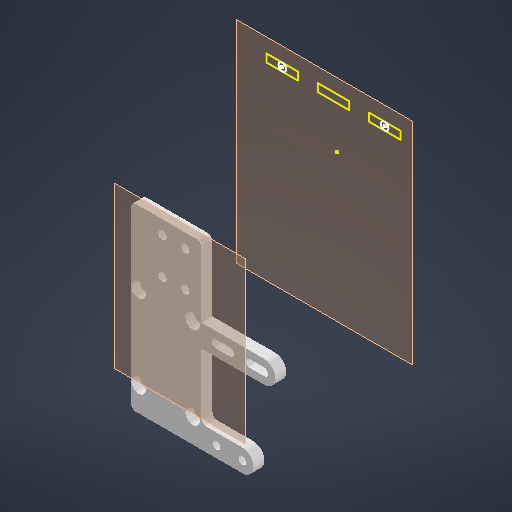
# Autodesk Inventor part: rails-bolts
Saved by Autodesk Inventor 2025 (Build 290162000, 162)
## iProperties
Created: 2024-07-18
Part Number: rails-bolts
Material: Generic
Document SubType Name: Modeling
Designer: Windows 7 was better
Density: 1 g/cm^3
Appearance: Default
Author: Windows 7 was better
Autodesk Inventor part; units mm, degrees
ref_plane "YZ Plane" through (0, 0, 0) normal (1, 0, 0) x (0, 1, 0)
ref_plane "XZ Plane" through (0, 0, 0) normal (0, 1, 0) x (-1, 0, 0)
ref_plane "XY Plane" through (0, 0, 0) normal (0, 0, 1) x (1, 0, 0)
ref_plane "Work Plane1" through (-1.6596, -28.9901, 28.1919) normal (0, 0, 1) x (1, 0, 0)
sketch "Sketch1" plane through (-1.6596, -28.9901, 28.1919) normal (0, 0, 1) x (1, 0, 0)
  circle A0 centre (-7.0449, 11.8967) radius 1.75 projected
  circle A1 centre (2.3051, 12.2717) radius 1.75 projected
  circle A2 centre (2.3051, 26.8467) radius 1.75 projected
  circle A3 centre (-7.0449, 26.8467) radius 1.75 projected
  line L0 (2.3051, 26.8467) -> (2.3051, 32.4467) construction
  line L1 (2.3051, 32.4467) -> (-7.0449, 32.4467) construction
  line L2 (-7.0449, 32.4467) -> (-7.0449, 26.8467) construction
  spline S0 degree 3 poles (-18.1261, -96.0287) (-18.1261, -96.0287) (-18.0932, -96.0287) (-18.0298, -96.0287) (-17.8251, -96.0287) (-17.2794, -96.0287) (-16.7467, -96.0287) (-16.213, -96.0287) (-15.7353, -96.0287) (-15.6244, -96.0287) (-15.6063, -96.0287) (-15.5971, -96.0287) (-15.5971, -96.0287) knots 0.499993 0.499993 0.499993 0.499993 0.562494 0.562494 0.562494 0.764477 0.764477 0.764477 0.966846 0.966846 0.966846 1 1 1 1 construction
  line L3 (-18.3185, -96.0287) -> (-15.9665, -96.0287) construction
  arc A4 (-13.8616, 2.5089) -> (-19.8616, 2.5089) centre (-16.8616, 2.5089) ccw construction
  arc A5 (-13.9993, -31.5037) -> (-19.9993, -31.5037) centre (-16.9993, -31.5037) ccw construction
  arc A6 (3.0015, -1.5044) -> (9.0015, -1.5044) centre (6.0015, -1.5044) ccw
  line L4 (-19.9993, 32.4467) -> (9.0007, 32.4467)
  line L5 (9.0007, 32.4467) -> (9.0007, -34.5533)
  line L6 (9.0007, -34.5533) -> (-19.9993, -34.5533)
  line L7 (-19.9993, -34.5533) -> (-19.9993, 32.4467)
  circle A7 centre (-16.8616, -31.5037) radius 1.6
  circle A8 centre (5.3371, -31.5037) radius 1.6
  circle A9 centre (-16.8616, 2.5089) radius 1.6
  circle A10 centre (5.3371, 2.5089) radius 1.6
  point P0 (1.6596, 28.9901)
  point P1 (-18.3185, 3.0171)
  point P2 (-15.9662, 3.4042)
  dimension "d0" = 5.6
  dimension "d1" = 29
  dimension "d2" = 67
  dimension "d5" = 3.2
  dimension "d6" = 3.2
  dimension "d7" = 3.2
  dimension "d8" = 3.2
  constraints: 16 end point, 7 centre point, 6 point on circle, 3 perpendicular, 2 horizontal, 2 parallel, 1 coincident, 1 vertical, 20 other
  measures "d0" distance of L0.start L0.end
  measures "d1" distance of L5.end L6.end
  measures "d2" distance of L4.end L5.end
  measures "d5" diameter of A7
  measures "d6" diameter of A8
  measures "d7" diameter of A9
  measures "d8" diameter of A10
ref_plane "Work Plane2" through (-8.6352, -23.8919, -35.0523) normal (0, 0, 1) x (1, 0, 0)
sketch "Sketch2" plane through (-8.6352, -23.8919, -35.0523) normal (0, 0, 1) x (1, 0, 0)
  line L0 (-7.5414, 41.3535) -> (-20.5414, 41.3535) projected
  line L1 (-20.5414, 44.5535) -> (-7.5414, 44.5535) projected
  line L2 (-7.5414, 44.5535) -> (-7.5414, 41.3535) projected
  line L3 (-20.5414, 41.3535) -> (-20.5414, 44.5535) projected
  line L4 (13.5, 41.3535) -> (0.5, 41.3535) projected
  line L5 (0.5, 44.5535) -> (13.5, 44.5535) projected
  line L6 (13.5, 44.5535) -> (13.5, 41.3535) projected
  line L7 (0.5, 41.3535) -> (0.5, 44.5535) projected
  line L8 (34.55, 41.3535) -> (21.55, 41.3535) projected
  line L9 (21.55, 44.5535) -> (34.55, 44.5535) projected
  line L10 (21.55, 41.3535) -> (21.55, 44.5535) projected
  line L11 (34.55, 44.5535) -> (34.55, 41.3535) projected
  line L12 (-14.0414, 44.5535) -> (-14.0414, 41.3535) construction
  line L13 (28.05, 44.5535) -> (28.05, 41.3535) construction
  circle A0 centre (-14.0414, 42.9535) radius 1.6
  circle A1 centre (28.05, 42.9535) radius 1.6
  point P0 (8.6352, 23.8919)
  constraints: 6 midpoint, 4 end point, 2 vertical alignment, 4 other
extrude "Extrusion1" add sketch "Sketch1" against normal blind 4.5
sketch "Sketch3" plane through (-1.6596, -28.9901, 28.1919) normal (0, 0, 1) x (1, 0, 0)
  line L0 (19.4071, -58.7998) -> (21.4071, -58.7998) construction
  line L1 (20.4071, -58.7998) -> (20.4979, -36.9098) construction
  line L2 (20.4979, -36.9098) -> (25.7879, -36.9098) construction
  line L3 (25.7879, -36.9098) -> (15.2079, -36.9098) construction
  circle A0 centre (15.2079, -36.9098) radius 1.6
  circle A1 centre (25.7879, -36.9098) radius 1.6
  circle A2 centre (15.2079, -36.9098) radius 4.6
  circle A3 centre (25.7879, -36.9098) radius 4.6
  line L4 (25.7879, -32.3098) -> (9.0007, -32.3098)
  line L5 (9.0007, -34.5533) -> (9.0007, 32.4467) projected
  line L6 (25.7879, -41.5098) -> (15.2079, -41.5098)
  line L7 (15.2079, -41.5098) -> (-19.9993, -41.5098)
  line L8 (-19.9993, -34.5533) -> (-19.9993, 32.4467) projected
  line L9 (-19.9993, -41.5098) -> (-19.9993, -34.5533)
  line L10 (-19.9993, -34.5533) -> (9.0007, -34.5533)
  line L11 (9.0007, -34.5533) -> (9.0007, -32.3098)
  line L12 (25.7879, -36.9098) -> (30.1497, -38.3706)
  line L13 (45.9071, 7.0963) -> (8.7371, 7.0963) construction
  line L14 (8.7371, 7.0963) -> (14.7371, 7.0963) construction
  line L15 (14.7371, 7.0963) -> (14.7371, -0.9037) construction
  line L16 (14.7371, -0.9037) -> (34.7371, -0.9037) construction
  line L17 (14.7371, -0.9037) -> (20.7371, -0.9037) construction
  line L18 (14.7371, -2.5037) -> (20.7371, -2.5037)
  line L19 (20.7371, 0.6963) -> (14.7371, 0.6963)
  arc A4 (14.7371, 0.6963) -> (14.7371, -2.5037) centre (14.7371, -0.9037) ccw
  arc A5 (20.7371, -2.5037) -> (20.7371, 0.6963) centre (20.7371, -0.9037) ccw
  line L20 (34.7371, -0.9037) -> (28.7371, -0.9037) construction
  line L21 (34.7371, 0.6963) -> (28.7371, 0.6963)
  line L22 (28.7371, -2.5037) -> (34.7371, -2.5037)
  arc A6 (34.7371, -2.5037) -> (34.7371, 0.6963) centre (34.7371, -0.9037) ccw
  arc A7 (28.7371, 0.6963) -> (28.7371, -2.5037) centre (28.7371, -0.9037) ccw
  line L23 (34.7371, 3.6963) -> (28.7371, 3.6963)
  arc A8 (28.7371, 3.6963) -> (28.7371, -5.5037) centre (28.7371, -0.9037) ccw
  line L24 (28.7371, -5.5037) -> (34.7371, -5.5037)
  arc A9 (34.7371, -5.5037) -> (34.7371, 3.6963) centre (34.7371, -0.9037) ccw
  line L25 (28.7371, 3.6963) -> (9.0007, 3.6963)
  line L26 (28.7371, -5.5037) -> (9.0007, -5.5037)
  point P0 (1.6596, 28.9901)
  point P1 (11.4479, -23.0098)
  point P2 (9.0007, -15.5098)
  point P3 (17.7371, -0.9037)
  point P4 (31.7371, -0.9037)
  dimension "d9" = 10.58
  dimension "d10" = 5.29
  dimension "d11" = 10.58
  dimension "d12" = 3.2
  dimension "d13" = 3.2
  dimension "d14" = 3
  dimension "d15" = 3
  dimension "d43" = 6
  dimension "d44" = 8
  dimension "d45" = 20
  dimension "d46" = 6
  dimension "d47" = 3.2
  dimension "d48" = 6
  dimension "d49" = 3.2
  dimension "d50" = 3
  constraints: 54 end point, 15 point on circle, 9 centre point, 9 tangent, 8 point on line, 7 perpendicular, 5 horizontal, 4 parallel, 3 midpoint, 2 coincident, 1 collinear, 1 vertical alignment, 12 other
  measures "d9" distance of L3.end L2.end
  measures "d10" distance of L1.end L2.end
  measures "d11" distance of L2.end L3.end
  measures "d12" diameter of A0
  measures "d13" diameter of A1
  measures "d15" radial gap between concentric circles of A1 A3
  measures "d43" distance of L13.end L14.end
  measures "d44" distance of L14.end L15.end
  measures "d45" distance of L15.end L16.end
  measures "d46" distance of L15.end L17.end
  measures "d47" diameter of A5
  measures "d48" distance of L16.end L20.end
  measures "d49" diameter of A7
  measures "d50" radial gap between concentric circles of A6 A9
extrude "Extrusion2" add sketch "Sketch3" against normal blind 4.5
sketch "Sketch4" plane through (-1.6596, -28.9901, 23.6919) normal (0, 0, -1) x (-1, 0, 0)
  circle A0 centre (-2.3051, 26.8467) radius 1.75 projected
  circle A1 centre (-2.3051, 26.8467) radius 3
  circle A2 centre (7.0449, 26.8467) radius 1.75 projected
  circle A3 centre (7.0449, 26.8467) radius 3
  circle A4 centre (-2.3051, 12.2165) radius 3
  circle A5 centre (7.0449, 11.8967) radius 1.75 projected
  circle A6 centre (7.0449, 11.8967) radius 3
  point P0 (-1.6596, 28.9901)
  dimension "d18" = 6
  dimension "d19" = 6
  dimension "d20" = 6
  dimension "d21" = 6
  constraints: 4 centre point, 3 coincident
  measures "d18" diameter of A1
  measures "d19" diameter of A3
  measures "d20" diameter of A4
  measures "d21" diameter of A6
extrude "Extrusion3" cut sketch "Sketch4" against normal blind 3 contours A1 | A2 | A3 | A4 | A6
fillet "Fillet1" radius 2 4 edges at (-21.6589, 3.4566, 25.9419) (-21.6589, -70.4999, 25.9419) (7.3411, -61.2999, 25.9419) (7.3411, 3.4566, 25.9419)
sketch "Sketch5" plane through (-1.6596, -28.9901, 28.1919) normal (0, 0, 1) x (1, 0, 0)
  circle A0 centre (-16.8616, 2.5089) radius 1.6 projected
  circle A1 centre (-16.8616, 2.5089) radius 3
  circle A2 centre (5.3371, 2.5089) radius 1.6 projected
  circle A3 centre (5.3371, 2.5089) radius 3
  circle A4 centre (-16.8616, -31.5037) radius 1.6 projected
  circle A5 centre (-16.8616, -31.5037) radius 3
  circle A6 centre (5.3371, -31.5037) radius 1.6 projected
  circle A7 centre (5.3371, -31.5037) radius 3
  point P0 (1.6596, 28.9901)
  dimension "d25" = 6
  dimension "d26" = 6
  dimension "d27" = 6
  dimension "d28" = 6
  constraints: 4 centre point, 4 coincident
  measures "d25" diameter of A1
  measures "d26" diameter of A3
  measures "d27" diameter of A5
  measures "d28" diameter of A7
extrude "Extrusion4" cut sketch "Sketch5" against normal blind 3.5 contours A1 | A2 | A3 | A5 | A7
body "Solid1"
